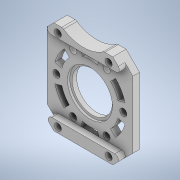
# Autodesk Inventor part: Versa Chassis Bearing Block
Saved by Autodesk Inventor 2020 (Build 240168000, 168)
## iProperties
Created: 2020-01-16
Part Number: Versa Chassis Bearing Block
Material: Generic
Document SubType Name: Modeling
Designer: aidan
Density: 1 g/cm^3
Appearance: Default
Author: aidan
Autodesk Inventor part; units mm, degrees
ref_plane "YZ Plane" through (0, 0, 0) normal (1, 0, 0) x (0, 1, 0)
ref_plane "XZ Plane" through (0, 0, 0) normal (0, 1, 0) x (-1, 0, 0)
ref_plane "XY Plane" through (0, 0, 0) normal (0, 0, 1) x (1, 0, 0)
sketch "Sketch2" plane through (0, 0, 0) normal (0, 0, 1) x (1, 0, 0)
  line L0 (-10.8368, 23.5104) -> (-10.8368, -29.6906) construction
  line L1 (-37.8996, -2.6413) -> (16.2259, -2.6413) construction
  circle A0 centre (-28.9216, 37.4694) radius 2.4892
  circle A1 centre (7.248, 37.4694) radius 2.4892
  circle A2 centre (-28.9216, -20.4172) radius 2.4892
  circle A3 centre (7.248, -20.4172) radius 2.4892
  line L2 (-28.9216, 37.4694) -> (7.248, 37.4694) construction
  line L3 (7.248, 37.4694) -> (7.248, -20.4172) construction
  line L4 (7.248, -20.4172) -> (-28.9216, -20.4172) construction
  line L5 (-28.9216, -20.4172) -> (-28.9216, 37.4694) construction
  line L6 (-41.3549, 42.4478) -> (19.6813, 42.4478)
  line L7 (19.6813, 42.4478) -> (19.6813, -24.2272)
  line L8 (19.6813, -24.2272) -> (-41.3549, -24.2272)
  line L9 (-41.3549, -24.2272) -> (-41.3549, 42.4478)
  line L10 (-10.8368, 42.4478) -> (-10.8368, -24.2272) construction
  point P0 (0, 0)
  point P1 (-10.8368, -2.6413)
  dimension "d9" = 36.1696
  dimension "d10" = 57.8866
  dimension "d11" = 4.9784
  dimension "d12" = 61.0362
  dimension "d13" = 66.675
  dimension "d15" = 3.81
  constraints: 22 end point, 4 centre point, 4 parallel, 3 equal radius, 3 horizontal, 3 midpoint, 3 perpendicular, 2 coincident, 1 collinear, 1 point on line, 1 other
  measures "d9" distance of L3.end L4.end
  measures "d10" distance of L2.end L3.end
  measures "d11" diameter of A0
  measures "d12" distance of L6.start L6.end
  measures "d13" distance of L6.end L7.end
  measures "d15" distance between parallel lines of L8 L4
extrude "Extrusion1" add sketch "Sketch2" along normal blind 9.525
sketch "Sketch3" plane through (0, 0, 9.525) normal (0, 0, 1) x (1, 0, 0)
  line L0 (-41.3549, 34.1928) -> (19.6813, 34.1928)
  line L1 (19.6813, 34.1928) -> (19.6813, -16.6072)
  line L2 (19.6813, -16.6072) -> (-41.3549, -16.6072)
  line L3 (-41.3549, -16.6072) -> (-41.3549, 34.1928)
  line L4 (19.6813, -24.2272) -> (19.6813, 42.4478) projected
  line L5 (-41.3549, 42.4478) -> (-41.3549, -24.2272) projected
  line L6 (-41.3549, -24.2272) -> (19.6813, -24.2272) projected
  point P0 (0, 0)
  dimension "d18" = 50.8
  dimension "d20" = 7.62
  constraints: 8 end point, 2 parallel, 2 point on line, 1 horizontal, 1 perpendicular
  measures "d18" distance of L0.end L1.end
  measures "d20" distance between parallel lines of L6 L2
extrude "Extrusion2" cut sketch "Sketch3" against normal blind 4.7498 contours L0 L1 L2 L3
chamfer "Chamfer1" distance 9.525 angle 45 4 edges at (19.6813, 42.4478, 4.7625) (-41.3549, 42.4478, 4.7625) (-41.3549, -24.2272, 4.7625) (19.6813, -24.2272, 4.7625)
fillet "Fillet1" radius 2.54 4 edges at (18.4113, 34.1928, 7.1501) (17.7763, -16.6072, 7.1501) (-39.4499, -16.6072, 7.1501) (-40.0849, 34.1928, 7.1501)
sketch "Sketch4" plane through (0, 0, 4.7752) normal (0, 0, 1) x (1, 0, 0)
  circle A0 centre (-10.8368, 7.2053) radius 14.2748
  line L0 (-41.3549, -14.7022) -> (-41.3549, 32.9228) projected
  line L1 (11.6442, -16.6072) -> (-33.3178, -16.6072) projected
  point P0 (0, 0)
  dimension "d27" = 30.5181
  dimension "d28" = 23.8125
  dimension "d29" = 28.5496
  constraints: 1 centre point
  measures "d27" distance from line of L0 A0.centre
  measures "d28" distance from line of L1 A0.centre
  measures "d29" diameter of A0
extrude "Extrusion3" cut sketch "Sketch4" against normal blind 4.7752
sketch "Sketch5" plane through (0, 0, 4.7752) normal (0, 0, 1) x (1, 0, 0)
  circle A0 centre (-10.8368, 7.2053) radius 14.2748 projected
  circle A1 centre (-10.8368, 7.2053) radius 15.9766
  point P0 (0, 0)
  dimension "d32" = 31.9532
  constraints: 1 centre point, 1 coincident
  measures "d32" diameter of A1
extrude "Extrusion4" cut sketch "Sketch5" against normal blind 1.6002
sketch "Sketch6" plane through (0, 0, 4.7752) normal (0, 0, 1) x (1, 0, 0)
  circle A0 centre (-10.8368, 7.2053) radius 14.2748 projected
  circle A1 centre (-10.8368, 7.2053) radius 14.2748 projected
  circle A2 centre (-10.8368, 7.2053) radius 23.8125 construction
  circle A3 centre (-34.6493, 7.2053) radius 2.4892
  point P0 (0, 0)
  dimension "d35" = 47.625
  dimension "d36" = 4.9784
  constraints: 1 centre point, 1 coincident, 1 horizontal alignment, 2 other
  measures "d36" diameter of A3
extrude "Extrusion5" cut sketch "Sketch6" against normal through all contours A3
pattern_circular "Circular Pattern1" count 6 over 360 about axis through (-10.8368, 7.2053, 4.7752) along (0, 0, -1) of "Extrusion5"
sketch "Sketch7" plane through (0, 0, 4.7752) normal (0, 0, 1) x (1, 0, 0)
  circle A0 centre (-10.8368, 7.2053) radius 14.2748 projected
  arc A1 (-5.4756, 27.2137) -> (-16.1981, 27.2137) centre (-10.8368, 7.2053) ccw
  arc A2 (-4.1608, 32.1206) -> (-17.5129, 32.1206) centre (-10.8368, 7.2053) ccw
  line L0 (-10.8368, 7.2053) -> (-10.8368, 32.9995) construction
  line L1 (-16.1981, 27.2137) -> (-17.5129, 32.1206)
  line L2 (-5.4756, 27.2137) -> (-4.1608, 32.1206)
  point P0 (0, 0)
  dimension "d42" = 5.08
  constraints: 6 end point, 5 point on circle, 2 centre point, 2 coincident, 1 vertical
  measures "d42" radial gap between concentric circles of A1 A2
extrude "Extrusion6" cut sketch "Sketch7" against normal through all contours A1 L1 A2 L2
pattern_circular "Circular Pattern2" count 6 over 360 about axis through (-10.8368, 7.2053, 4.7752) along (0, 0, -1) of "Extrusion6"
sketch "Sketch8" plane through (0, 0, 9.525) normal (0, 0, 1) x (1, 0, 0)
  line L0 (10.1563, 42.4478) -> (-31.8299, 42.4478) projected
  arc A0 (-25.4799, 42.4478) -> (3.8063, 42.4478) centre (-10.8368, 63.2021) ccw
  point P0 (0, 0)
  dimension "d49" = 6.35
  dimension "d50" = 6.35
  dimension "d51" = 25.4
  constraints: 2 point on circle, 2 point on line, 1 centre point
  measures "d49" distance of L0.end A0.start
  measures "d50" distance of L0.start A0.end
  measures "d51" radius of A0
extrude "Extrusion7" cut sketch "Sketch8" against normal through all
fillet "Fillet2" radius 2.54 2 edges at (-25.4799, 42.4478, 4.7625) (3.8063, 42.4478, 4.7625)
equation "\"d15\" = d14"
equation "\"d20\" = d19"
equation "\"d14\" = 3.81"
equation "\"d19\" = 2 * d14"
body "Solid1"
